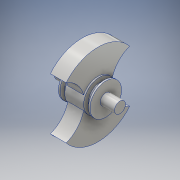
# Autodesk Inventor part: arma
Saved by Autodesk Inventor 2016 (Build 200138000, 138)
## iProperties
Created: 2019-03-15
Part Number: arma
Material: Aluminio 6061
Document SubType Name: Modeling
Designer: FIMCP
Density: 2.7 g/cm^3
Appearance: Aluminio - Plano
Mass: 33.1655 g
Surface Area: 49.4921 cm^2
Volume: 12.2835 cm^3
Author: FIMCP
Autodesk Inventor part; units mm, degrees
ref_plane "YZ Plane" through (0, 0, 0) normal (1, 0, 0) x (0, 1, 0)
ref_plane "XZ Plane" through (0, 0, 0) normal (0, 1, 0) x (-1, 0, 0)
ref_plane "XY Plane" through (0, 0, 0) normal (0, 0, 1) x (1, 0, 0)
sketch "Boceto1" plane through (0, 0, 0) normal (1, 0, 0) x (0, 1, 0)
  circle A0 centre (0, 0) radius 3.5
  dimension "d0" = 7
  constraints: 1 centre point, 1 coincident
  measures "d0" diameter of A0
extrude "Extrusión1" add sketch "Boceto1" along normal mid plane 38
sketch "Boceto2" plane through (0, 0, 0) normal (1, 0, 0) x (0, 1, 0)
  arc A0 (20.1106, 16.4792) -> (20.1106, -16.4792) centre (26, 0) ccw
  arc A1 (-20.1106, -16.4792) -> (-20.1106, 16.4792) centre (-26, 0) ccw
  arc A2 (-20.1106, -16.4792) -> (20.1106, -16.4792) centre (0, 0) ccw
  arc A3 (20.1106, 16.4792) -> (-20.1106, 16.4792) centre (0, 0) ccw
  dimension "d22" = 35
  dimension "d23" = 35
  constraints: 8 point on circle, 4 centre point
  measures "d22" diameter of A0
  measures "d23" diameter of A1
extrude "Extrusión2" add sketch "Boceto2" along normal mid plane 10
sketch "Boceto3" plane through (0, 0, 0) normal (1, 0, 0) x (0, 1, 0)
  circle A0 centre (0, 0) radius 10
  dimension "d8" = 20
  constraints: 1 centre point, 1 coincident
  measures "d8" diameter of A0
extrude "Extrusión3" add sketch "Boceto3" along normal mid plane 12
sketch "Boceto4" plane through (0, 0, 0) normal (1, 0, 0) x (0, 1, 0)
  circle A0 centre (0, 0) radius 3.5 projected
  circle A1 centre (0, 0) radius 7
  dimension "d11" = 14
  constraints: 1 centre point, 1 coincident
  measures "d11" diameter of A1
extrude "Extrusión4" add sketch "Boceto4" along normal mid plane 20
sketch "Boceto6" plane through (0, 0, 0) normal (0, 1, 0) x (-1, 0, 0)
  line L0 (10, -3.5) -> (10, 3.5) projected
  line L1 (10, 0) -> (9, 0)
  line L2 (9, 0) -> (9, -10)
  line L3 (9, -10) -> (10, -10)
  line L4 (10, -10) -> (10, 0)
  line L5 (26.6, 0) -> (-26.6, 0) projected
  point P0 (0, 0)
  dimension "d15" = 1
  dimension "d16" = 10
  constraints: 8 end point, 2 parallel, 1 horizontal, 1 midpoint, 1 perpendicular
  measures "d15" distance of L3.end L2.end
  measures "d16" distance of L2.end L1.end
revolve "Revolución1" add sketch "Boceto6" angle 360 about axis through (-10, 0, 0) along (1, 0, 0)
sketch "Boceto7" plane through (0, 0, 0) normal (0, 1, 0) x (-1, 0, 0)
  line L0 (-10, 7) -> (-10, -7) projected
  line L1 (-10, 0) -> (-9, 0)
  line L2 (-9, 0) -> (-9, -10)
  line L3 (-9, -10) -> (-10, -10)
  line L4 (-10, -10) -> (-10, 0)
  line L5 (26.6, 0) -> (-26.6, 0) projected
  point P0 (0, 0)
  dimension "d18" = 1
  dimension "d19" = 10
  constraints: 8 end point, 2 parallel, 1 horizontal, 1 midpoint, 1 perpendicular
  measures "d18" distance of L2.end L3.end
  measures "d19" distance of L1.end L2.end
revolve "Revolución2" add sketch "Boceto7" angle 360 about axis through (-10, 0, 0) along (1, 0, 0)
